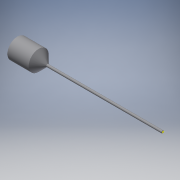
# Autodesk Inventor part: Drill 8
Saved by Autodesk Inventor 2018 (Build 220112000, 112)
## iProperties
Created: 2021-03-25
Part Number: Drill 8
Material: Generic
Document SubType Name: Modeling
Designer: Charles.Rymal
Density: 1 g/cm^3
Appearance: Default
Author: Charles.Rymal
Autodesk Inventor part; units mm, degrees
ref_plane "YZ Plane" through (0, 0, 0) normal (1, 0, 0) x (0, 1, 0)
ref_plane "XZ Plane" through (0, 0, 0) normal (0, 1, 0) x (-1, 0, 0)
ref_plane "XY Plane" through (0, 0, 0) normal (0, 0, 1) x (1, 0, 0)
sketch "Sketch1" plane through (0, 0, 0) normal (0, 0, 1) x (1, 0, 0)
  line L0 (-13.8928, 3.175) -> (278.2072, 3.175)
  line L1 (278.2072, 3.175) -> (278.2072, 0)
  line L2 (278.2072, 0) -> (0, 0)
  line L3 (0, 0) -> (-90.0928, 0)
  line L4 (-90.0928, 0) -> (-90.0928, 25.4)
  line L5 (-90.0928, 25.4) -> (-13.8928, 25.4)
  line L6 (-13.8928, 25.4) -> (-13.8928, 3.175)
  line L7 (-13.8928, 3.175) -> (-36.1178, 25.4)
  dimension "d0" = 3.175
  dimension "d1" = 292.1
  dimension "d2" = 25.4
  dimension "d3" = 76.2
  dimension "d5" = 45
  constraints: 17 end point, 5 perpendicular, 2 point on line, 1 horizontal
  measures "d0" distance between parallel lines of L2 L0
  measures "d1" distance of L0.start L0.end
  measures "d2" distance between parallel lines of L3 L5
  measures "d3" distance of L4.end L5.end
  measures "d5" angle of L6 L7
revolve "Revolution1" add sketch "Sketch1" angle 360 about axis through (0, 0, 0) along (-1, 0, 0) contours L0 L1 L2 L3 L4 L5 L7
body "Solid1"
